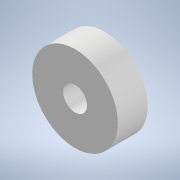
# Autodesk Inventor part: rodamiento_carril
Saved by Autodesk Inventor 2022 (Build 260153000, 153)
## iProperties
Created: 2022-03-05
Part Number: rodamiento_carril
Material: Generic
Document SubType Name: Modeling
Designer: katha
Density: 1 g/cm^3
Appearance: Default
Author: katha
Autodesk Inventor part; units mm, degrees
ref_plane "YZ Plane" through (0, 0, 0) normal (1, 0, 0) x (0, 1, 0)
ref_plane "XZ Plane" through (0, 0, 0) normal (0, 1, 0) x (-1, 0, 0)
ref_plane "XY Plane" through (0, 0, 0) normal (0, 0, 1) x (1, 0, 0)
sketch "Sketch1" plane through (0, 0, 0) normal (0, 0, 1) x (1, 0, 0)
  circle A0 centre (15, 0) radius 2.5 projected
  circle A1 centre (15, 0) radius 3
  circle A2 centre (15, 0) radius 10.75
  point P0 (0, 0)
  dimension "d0" = 6
  dimension "d1" = 21.5
  constraints: 2 centre point, 2 coincident
  measures "d0" diameter of A1
  measures "d1" diameter of A2
extrude "Extrusion1" add sketch "Sketch1" against normal blind 7.5 contours A2
body "Solid1"
